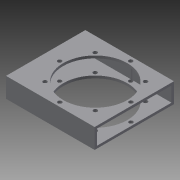
# Autodesk Inventor part: 4x1x5 box beam
Saved by Autodesk Inventor 2015 (Build 190159000, 159)
## iProperties
Created: 2015-02-14
Part Number: 4x1x5 box beam
Material: Generic
Document SubType Name: Modeling
Designer: chapale16
Density: 1 g/cm^3
Appearance: Default
Author: chapale16
Autodesk Inventor part; units mm, degrees
ref_plane "YZ Plane" through (0, 0, 0) normal (1, 0, 0) x (0, 1, 0)
ref_plane "XZ Plane" through (0, 0, 0) normal (0, 1, 0) x (-1, 0, 0)
ref_plane "XY Plane" through (0, 0, 0) normal (0, 0, 1) x (1, 0, 0)
sketch "Sketch1" plane through (0, 0, 0) normal (1, 0, 0) x (0, 1, 0)
  line L0 (0, 0) -> (-25.4, 0)
  line L1 (-25.4, 0) -> (-25.4, -101.6)
  line L2 (-25.4, -101.6) -> (0, -101.6)
  line L3 (0, -101.6) -> (0, 0)
  line L4 (-3.175, -3.175) -> (-22.225, -3.175)
  line L5 (-22.225, -3.175) -> (-22.225, -98.425)
  line L6 (-22.225, -98.425) -> (-3.175, -98.425)
  line L7 (-3.175, -98.425) -> (-3.175, -3.175)
  dimension "d0" = 25.4
  dimension "d1" = 101.6
  dimension "d2" = 3.175
  constraints: 16 end point, 4 parallel, 2 perpendicular, 1 horizontal, 3 other
  measures "d0" distance of L2.end L1.end
  measures "d1" distance of L1.end L0.end
  measures "d2" distance between parallel lines of L3 L7
extrude "Extrusion1" add sketch "Sketch1" along normal blind 127
sketch "Sketch2" plane through (0, 0, 0) normal (0, 1, 0) x (1, 0, 0)
  circle A0 centre (63.5, 50.8) radius 41 projected
  point P0 (0, 0)
extrude "Extrusion2" cut sketch "Sketch2" against normal blind 127
sketch "Sketch3" plane through (0, 0, 0) normal (0, 1, 0) x (1, 0, 0)
  circle A0 centre (63.5, 50.8) radius 49.5 projected
  circle A1 centre (31.251, 82.8975) radius 2.55 projected
  circle A2 centre (63.3929, 96.2999) radius 2.55 projected
  circle A3 centre (95.5975, 83.049) radius 2.55 projected
  circle A4 centre (108.9999, 50.9071) radius 2.55 projected
  circle A5 centre (95.749, 18.7025) radius 2.55 projected
  circle A6 centre (63.6071, 5.3001) radius 2.55 projected
  circle A7 centre (31.4025, 18.551) radius 2.55 projected
  circle A8 centre (18.0001, 50.6929) radius 2.55 projected
  circle A9 centre (63.5, 50.8) radius 29 projected
  point P0 (0, 0)
extrude "Extrusion3" cut sketch "Sketch3" against normal blind 127 contours A1 | A2 | A3 | A4 | A5 | A6 | A7 | A8
sketch "Sketch4" plane through (0, 0, 0) normal (0, 1, 0) x (1, 0, 0)
  circle A0 centre (31.4025, 18.551) radius 2.55 projected
  circle A1 centre (95.749, 18.7025) radius 2.55 projected
  circle A2 centre (95.5975, 83.049) radius 2.55 projected
  circle A3 centre (31.251, 82.8975) radius 2.55 projected
  circle A4 centre (63.3929, 96.2999) radius 2.55 projected
  circle A5 centre (108.9999, 50.9071) radius 2.55 projected
  circle A6 centre (63.6071, 5.3001) radius 2.55 projected
  circle A7 centre (18.0001, 50.6929) radius 2.55 projected
  circle A8 centre (63.5, 50.8) radius 41 projected
  line L0 (0, 101.6) -> (0, 0) projected
  line L1 (0, 0) -> (127, 0) projected
  line L2 (127, 101.6) -> (127, 0) projected
  line L3 (0, 101.6) -> (127, 101.6) projected
  line L4 (0, 101.6) -> (127, 101.6) projected
  line L5 (127, 0) -> (113.4618, 0)
  line L6 (113.4618, 0) -> (113.4618, 101.6)
  line L7 (113.4618, 101.6) -> (127, 101.6)
  line L8 (127, 101.6) -> (127, 0)
  dimension "d9" = 13.5382
  constraints: 8 end point, 2 parallel, 1 horizontal, 1 perpendicular, 1 point on line
  measures "d9" distance of L6.end L7.end
extrude "Extrusion4" cut sketch "Sketch4" against normal blind 127 contours L3 L2 L1 L6
sketch "Sketch6" plane through (0, 0, 0) normal (0, 1, 0) x (1, 0, 0)
  circle A0 centre (10.2546, 88.1171) radius 3.175 projected
  circle A1 centre (-15.1454, 88.2911) radius 3.175 projected
  arc A2 (59.2572, 91.5755) -> (37.6675, 82.6327) centre (63.5, 50.8) ccw projected
  arc A3 (58.9842, 100.7643) -> (59.2572, 91.5755) centre (63.5, 96.3) ccw projected
  line L0 (-60.4471, 100.7643) -> (58.9842, 100.7643) projected
  line L1 (-60.4471, 100.7643) -> (-35.0471, 75.3643) projected
  line L2 (-35.0471, 75.3643) -> (30.6788, 75.3643) projected
  arc A4 (31.6673, 76.6325) -> (30.6788, 75.3643) centre (63.5, 50.8) ccw projected
  arc A5 (37.6675, 82.6327) -> (31.6673, 76.6325) centre (31.3266, 82.9734) ccw projected
  circle A6 centre (63.5, 50.8) radius 9.525 projected
  circle A7 centre (-15.1454, 88.2911) radius 3.175 projected
  circle A8 centre (100.7643, -2.7658) radius 3.175 projected
  circle A9 centre (10.2546, 88.1171) radius 3.175 projected
  line L3 (113.4643, 100.7643) -> (113.4643, -13.5357) projected
  line L4 (-35.8911, 100.7643) -> (113.4643, 100.7643) projected
  line L5 (-35.8911, 100.7643) -> (-4.2078, -13.5357) projected
  line L6 (113.4643, -13.5357) -> (-4.2078, -13.5357) projected
  arc A10 (91.2393, 44.7826) -> (91.2393, 56.8174) centre (63.5, 50.8) ccw projected
  line L7 (91.2393, -13.5357) -> (91.2393, 44.7826) projected
  line L8 (110.2893, -13.5357) -> (91.2393, -13.5357) projected
  line L9 (110.2893, -13.5357) -> (110.2893, 100.7643) projected
  line L10 (91.2393, 100.7643) -> (110.2893, 100.7643) projected
  line L11 (91.2393, 56.8174) -> (91.2393, 100.7643) projected
  line L12 (113.4618, 0) -> (113.4618, 101.6) projected
  line L13 (0, 101.6) -> (113.4618, 101.6) projected
  line L14 (0, 101.6) -> (0, 0) projected
  line L15 (0, 0) -> (113.4618, 0) projected
  circle A11 centre (63.5, 50.8) radius 41 projected
  circle A12 centre (18.0001, 50.6929) radius 2.55 projected
  circle A13 centre (63.6071, 5.3001) radius 2.55 projected
  circle A14 centre (108.9999, 50.9071) radius 2.55 projected
  circle A15 centre (63.3929, 96.2999) radius 2.55 projected
  circle A16 centre (31.251, 82.8975) radius 2.55 projected
  circle A17 centre (95.5975, 83.049) radius 2.55 projected
  circle A18 centre (95.749, 18.7025) radius 2.55 projected
  circle A19 centre (31.4025, 18.551) radius 2.55 projected
  circle A20 centre (100.7643, 9.8) radius 3.175
  circle A21 centre (10.2546, 9.8) radius 3.175
  circle A22 centre (100.7643, 91.8) radius 3.175
  circle A23 centre (10.2546, 9.8) radius 3.175 projected
  circle A24 centre (100.7643, 9.8) radius 3.175 projected
  circle A25 centre (100.7643, 91.8) radius 3.175 projected
  dimension "d12" = 6.35
  dimension "d13" = 6.35
  dimension "d14" = 6.35
  constraints: 3 centre point
  measures "d12" diameter of A20
  measures "d13" diameter of A21
  measures "d14" diameter of A22
extrude "Extrusion5" cut sketch "Sketch6" against normal blind 127 contours A0 | A20 | A21 | A22
body "Solid1"
